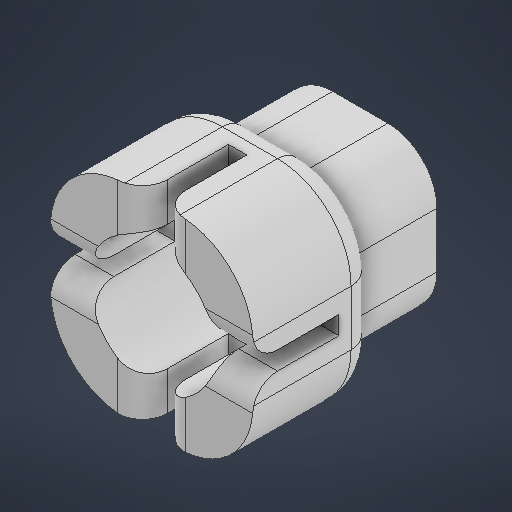
# Autodesk Inventor part: adapter-02
Saved by Autodesk Inventor 2026 (Build 300175050, 175E)
## iProperties
Created: 2025-05-28
Part Number: adapter-02
Material: Generic
Document SubType Name: Modeling
Designer: aduwa
Density: 1 g/cm^3
Appearance: Default
Author: aduwa
Autodesk Inventor part; units mm, degrees
ref_plane "YZ Plane" through (0, 0, 0) normal (1, 0, 0) x (0, 1, 0)
ref_plane "XZ Plane" through (0, 0, 0) normal (0, 1, 0) x (-1, 0, 0)
ref_plane "XY Plane" through (0, 0, 0) normal (0, 0, 1) x (1, 0, 0)
sketch "Sketch1" plane through (0, 0, 0) normal (0, 0, 1) x (1, 0, 0)
  circle A0 centre (0, 0) radius 5.15
  line L0 (-8.25, 8.25) -> (8.25, 8.25)
  line L1 (8.25, 8.25) -> (8.25, -8.25)
  line L2 (8.25, -8.25) -> (-8.25, -8.25)
  line L3 (-8.25, -8.25) -> (-8.25, 8.25)
  line L4 (-8.25, 8.25) -> (8.25, -8.25) construction
  line L5 (8.25, 8.25) -> (-8.25, -8.25) construction
  line L6 (0.75, -8.25) -> (-0.75, -8.25)
  line L7 (-0.75, -8.25) -> (-0.75, 8.25)
  line L8 (-0.75, 8.25) -> (0.75, 8.25)
  line L9 (0.75, 8.25) -> (0.75, -8.25)
  line L10 (0.75, -8.25) -> (-0.75, 8.25) construction
  line L11 (-0.75, -8.25) -> (0.75, 8.25) construction
  line L12 (8.25, 0.75) -> (-8.25, 0.75)
  line L13 (-8.25, 0.75) -> (-8.25, -0.75)
  line L14 (-8.25, -0.75) -> (8.25, -0.75)
  line L15 (8.25, -0.75) -> (8.25, 0.75)
  line L16 (8.25, 0.75) -> (-8.25, -0.75) construction
  line L17 (-8.25, 0.75) -> (8.25, -0.75) construction
  point P0 (2.2177, -5.7994)
  point P1 (6.5123, -1.5048)
  point P2 (9.7177, -1.5048)
  point P3 (9.7177, -0.0048)
  point P4 (6.5123, -0.0048)
  point P5 (2.2177, 4.2897)
  point P6 (2.2177, 7.4952)
  point P7 (0.7177, 4.2897)
  point P8 (-3.5768, -0.0048)
  point P9 (-6.7823, -0.0048)
  point P10 (-3.5768, -1.5048)
  point P11 (0.7177, -5.7994)
  point P12 (0.7177, -9.0048)
  point P13 (2.2177, -9.0048)
  point P14 (0.75, -5.0951)
  point P15 (-0.75, -5.0951)
  point P16 (5.0951, -0.75)
  point P17 (5.0951, 0.75)
  point P18 (-5.0951, -0.75)
  point P19 (-5.0951, 0.75)
  point P20 (0.75, 5.0951)
  point P21 (-0.75, 5.0951)
  dimension "d0" = 10.3
  dimension "d1" = 16.5
  dimension "d2" = 1.5
  dimension "d3" = 1.5
  dimension "d4" = 16.5
  constraints: 36 end point, 6 midpoint, 6 parallel, 3 horizontal, 3 perpendicular, 2 point on line, 1 centre point, 1 coincident
  measures "d0" diameter of A0
  measures "d1" distance of L1.end L2.end
  measures "d2" distance of L7.end L8.end
  measures "d3" distance of L13.end L12.end
  measures "d4" distance of L0.end L1.end
extrude "face" add sketch "Sketch1" against normal blind 10 contours A0 L12 L1 L14 | A0 L9 L0 L1 L12 | L14 L1 L2 L9 A0 | A0 L7 L0 L9 | L9 L2 L7 A0 | A0 L12 L3 L0 L7 | L7 L2 L3 L14 A0 | A0 L14 L3 L12
extrude "Extrusion2" cut sketch "Sketch1" against normal blind 7 contours A0 L12 L1 L14 | A0 L7 L0 L9 | L9 L2 L7 A0 | A0 L14 L3 L12
fillet "Fillet1" radius 6 4 edges at (-8.25, 8.25, -5) (8.25, -8.25, -5) (8.25, 8.25, -5) (-8.25, -8.25, -5)
fillet "Fillet2" radius 2 8 edges at (-8.25, 0, -10) (-6.4926, -6.4926, -10) (0, -8.25, -10) (6.4926, -6.4926, -10) (8.25, 0, -10) (6.4926, 6.4926, -10) (0, 8.25, -10) (-6.4926, 6.4926, -10)
fillet "Fillet4" radius 2 8 edges at (0.75, -6.6725, 0) (-0.75, -6.6725, 0) (-6.6725, -0.75, 0) (-6.6725, 0.75, 0) (-0.75, 6.6725, 0) (0.75, 6.6725, 0) (6.6725, 0.75, 0) (6.6725, -0.75, 0)
sketch "Sketch6" plane through (0, 0, -10) normal (0, 0, -1) x (-1, 0, 0)
  circle A0 centre (0, 0) radius 5.15 projected
  line L0 (6.25, 2.25) -> (6.25, -2.25) projected
  arc A1 (6.25, 2.25) -> (2.25, 6.25) centre (2.25, 2.25) ccw projected
  line L1 (-2.25, 6.25) -> (2.25, 6.25) projected
  arc A2 (-2.25, 6.25) -> (-6.25, 2.25) centre (-2.25, 2.25) ccw projected
  line L2 (-6.25, -2.25) -> (-6.25, 2.25) projected
  arc A3 (-6.25, -2.25) -> (-2.25, -6.25) centre (-2.25, -2.25) ccw projected
  line L3 (2.25, -6.25) -> (-2.25, -6.25) projected
  arc A4 (2.25, -6.25) -> (6.25, -2.25) centre (2.25, -2.25) ccw projected
extrude "Extrusion9" add sketch "Sketch6" along normal blind 7 contours A0 | L0 A4 L3 A3 L2 A2 L1 A1
sketch "Sketch7" plane through (0, 0, -17) normal (0, 0, -1) x (-1, 0, 0)
  line L0 (4.5207, 0) -> (2.2603, -3.915)
  line L1 (2.2603, -3.915) -> (-2.2603, -3.915)
  line L2 (-2.2603, -3.915) -> (-4.5207, 0)
  line L3 (-4.5207, 0) -> (-2.2603, 3.915)
  line L4 (-2.2603, 3.915) -> (2.2603, 3.915)
  line L5 (2.2603, 3.915) -> (4.5207, 0)
  line L6 (2.3758, -4.115) -> (4.7516, 0)
  line L7 (4.7516, 0) -> (2.3758, 4.115)
  line L8 (2.3758, 4.115) -> (-2.3758, 4.115)
  line L9 (-2.3758, 4.115) -> (-4.7516, 0)
  line L10 (-4.7516, 0) -> (-2.3758, -4.115)
  line L11 (-2.3758, -4.115) -> (2.3758, -4.115)
  circle A0 centre (0, 0) radius 3.5
  dimension "d34" = 7.83
  dimension "d35" = 0.2
  dimension "d38" = 7
  constraints: 24 end point, 2 coincident, 1 centre point, 18 other
  measures "d34" distance between parallel lines of L4 L1
  measures "d35" distance between parallel lines of L0 L6
  measures "d38" diameter of A0
extrude "Extrusion10" cut sketch "Sketch7" against normal blind 3.5 contours L0 L1 L2 L3 L4 L5 | L11 L10 L9 L8 L7 L6 | A0
sketch "Sketch8" plane through (0, 0, -10) normal (0, 0, 1) x (1, 0, 0)
  line L0 (4.5207, 0) -> (2.2603, -3.915)
  line L1 (2.2603, -3.915) -> (-2.2603, -3.915)
  line L2 (-2.2603, -3.915) -> (-4.5207, 0)
  line L3 (-4.5207, 0) -> (-2.2603, 3.915)
  line L4 (-2.2603, 3.915) -> (2.2603, 3.915)
  line L5 (2.2603, 3.915) -> (4.5207, 0)
  line L6 (2.4335, -4.215) -> (4.8671, 0)
  line L7 (4.8671, 0) -> (2.4335, 4.215)
  line L8 (2.4335, 4.215) -> (-2.4335, 4.215)
  line L9 (-2.4335, 4.215) -> (-4.8671, 0)
  line L10 (-4.8671, 0) -> (-2.4335, -4.215)
  line L11 (-2.4335, -4.215) -> (2.4335, -4.215)
  circle A0 centre (0, 0) radius 3.5
  dimension "d41" = 7.83
  dimension "d42" = 0.3
  dimension "d43" = 7
  constraints: 24 end point, 3 coincident, 1 centre point, 18 other
  measures "d41" distance between parallel lines of L4 L1
  measures "d42" distance between parallel lines of L0 L6
  measures "d43" diameter of A0
extrude "Extrusion12" [suppressed]
sketch "Sketch9" plane through (0, 0, -17) normal (0, 0, -1) x (-1, 0, 0)
  circle A0 centre (0, 0) radius 2.6
  circle A1 centre (0, 0) radius 4
  dimension "d46" = 5.2
  dimension "d47" = 8
  constraints: 2 centre point, 2 coincident
  measures "d46" diameter of A0
  measures "d47" diameter of A1
extrude "Extrusion13" [suppressed]
extrude "Extrusion14" [suppressed]
body "Solid1"
